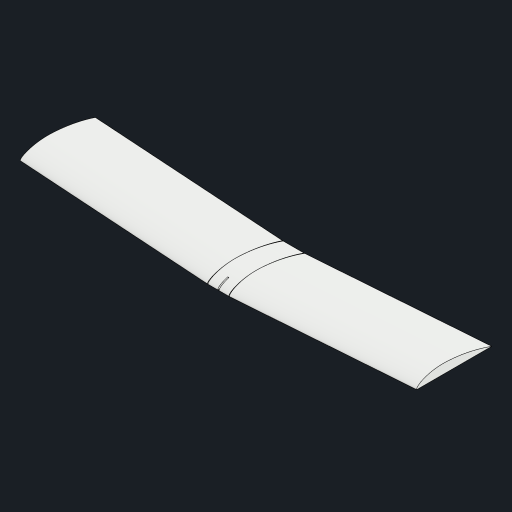
# Autodesk Inventor part: MainWing
Saved by Autodesk Inventor 2023 (Build 270158000, 158)
## iProperties
Created: 2022-05-12
Part Number: MainWing
Material: カインズの発泡スチロール
Document SubType Name: Modeling
Designer: neko2
Density: 0.02 g/cm^3
Appearance: 一般
Mass: 50.154 g
Surface Area: 3566.31 cm^2
Volume: 2507.7 cm^3
Author: neko2
Autodesk Inventor part; units mm, degrees
ref_plane "YZ Plane" through (0, 0, 0) normal (1, 0, 0) x (0, 1, 0)
ref_plane "XZ Plane" through (0, 0, 0) normal (0, 1, 0) x (-1, 0, 0)
ref_plane "XY Plane" through (0, 0, 0) normal (0, 0, 1) x (1, 0, 0)
sketch "スケッチ1" plane through (0, 0, 0) normal (1, 0, 0) x (0, 1, 0)
  spline S0 degree 3 poles (0, 0) (0.6026, 0.1485) (1.1749, 0.124) (1.7185, -0.0273) (2.4135, -0.2207) (3.0615, -0.6212) (3.65, -1.0753) (4.4423, -1.6866) (5.1266, -2.395) (5.7619, -3.1474) (6.5814, -4.1179) (7.3194, -5.1616) (8.0039, -6.2364) (8.8443, -7.5561) (9.6039, -8.9229) (10.3094, -10.317) (11.1425, -11.9631) (11.9, -13.6474) (12.5994, -15.355) (13.3997, -17.3089) (14.1237, -19.2933) (14.7857, -21.298) (15.5246, -23.5358) (16.1861, -25.7989) (16.7802, -28.0794) (17.4299, -30.5737) (17.9989, -33.0887) (18.4948, -35.618) (19.0279, -38.3372) (19.4765, -41.0727) (19.8487, -43.8185) (20.2428, -46.7262) (20.5512, -49.6454) (20.779, -52.5708) (21.0171, -55.6293) (21.1671, -58.6947) (21.2319, -61.7617) (21.2988, -64.9292) (21.2748, -68.0985) (21.1769, -71.265) (21.079, -74.4325) (20.9071, -77.5972) (20.6919, -80.7589) (20.4747, -83.9491) (20.2135, -87.1362) (19.9062, -90.3189) (19.5988, -93.503) (19.2453, -96.6827) (18.8489, -99.857) (18.4567, -102.9968) (18.0225, -106.1313) (17.5487, -109.2598) (17.0852, -112.3209) (16.5839, -115.3762) (16.0455, -118.4249) (15.525, -121.3728) (14.9697, -124.3146) (14.3808, -127.2496) (13.8184, -130.0529) (13.2253, -132.8499) (12.6033, -135.6405) (12.0172, -138.2695) (11.4054, -140.8927) (10.767, -143.5095) (10.1749, -145.936) (9.5598, -148.3569) (8.9224, -150.772) (8.342, -152.9711) (7.7431, -155.1653) (7.1255, -157.3543) (6.5752, -159.305) (6.0101, -161.2514) (5.4303, -163.1935) (4.9282, -164.8752) (4.4152, -166.5537) (3.8908, -168.2286) (3.4532, -169.6264) (3.0078, -171.0218) (2.554, -172.4145) (2.1955, -173.5145) (1.8319, -174.6128) (1.4648, -175.7099) (1.1994, -176.5028) (0.9323, -177.2952) (0.661, -178.0861) (0.497, -178.5643) (0.3315, -179.042) (0.1662, -179.5197) (0.1108, -179.6798) (0.0554, -179.8399) (0, -180) knots -1.050464 -1.050464 -1.050464 -1.050464 -1.040913 -1.040913 -1.040913 -1.028702 -1.028702 -1.028702 -1.012261 -1.012261 -1.012261 -0.991051 -0.991051 -0.991051 -0.965006 -0.965006 -0.965006 -0.934253 -0.934253 -0.934253 -0.899065 -0.899065 -0.899065 -0.859785 -0.859785 -0.859785 -0.816823 -0.816823 -0.816823 -0.770637 -0.770637 -0.770637 -0.721726 -0.721726 -0.721726 -0.670591 -0.670591 -0.670591 -0.617781 -0.617781 -0.617781 -0.564955 -0.564955 -0.564955 -0.511651 -0.511651 -0.511651 -0.458324 -0.458324 -0.458324 -0.405576 -0.405576 -0.405576 -0.353966 -0.353966 -0.353966 -0.304062 -0.304062 -0.304062 -0.2564 -0.2564 -0.2564 -0.211497 -0.211497 -0.211497 -0.169859 -0.169859 -0.169859 -0.131943 -0.131943 -0.131943 -0.098154 -0.098154 -0.098154 -0.068896 -0.068896 -0.068896 -0.044478 -0.044478 -0.044478 -0.025191 -0.025191 -0.025191 -0.011252 -0.011252 -0.011252 -0.002824 -0.002824 -0.002824 0 0 0 0
  spline S1 degree 3 poles (0, -180) (-0.1069, -180.01) (-0.1817, -179.9953) (-0.2232, -179.955) (-0.3155, -179.8653) (-0.2429, -179.6486) (-0.1926, -179.4492) (-0.0424, -178.853) (-0.0927, -178.4107) (-0.1026, -177.9372) (-0.1189, -177.1543) (-0.0246, -176.2861) (0.0432, -175.437) (0.1368, -174.2642) (0.1798, -173.1279) (0.2322, -171.9828) (0.2984, -170.5361) (0.3796, -169.0753) (0.4536, -167.6178) (0.5421, -165.8746) (0.6202, -164.136) (0.6948, -162.396) (0.7808, -160.392) (0.8622, -158.3861) (0.936, -156.3804) (1.0186, -154.1358) (1.0916, -151.8914) (1.1574, -149.6466) (1.2294, -147.1881) (1.2927, -144.7293) (1.3446, -142.2702) (1.4004, -139.6274) (1.4429, -136.9844) (1.4742, -134.3412) (1.5073, -131.5441) (1.5278, -128.7469) (1.5354, -125.9496) (1.5433, -123.0294) (1.5371, -120.1091) (1.5174, -117.189) (1.4971, -114.1787) (1.4624, -111.1684) (1.4148, -108.1584) (1.3663, -105.091) (1.3045, -102.0237) (1.2312, -98.9568) (1.1574, -95.8653) (1.0719, -92.7741) (0.9756, -89.6832) (0.8795, -86.5996) (0.7725, -83.5163) (0.666, -80.433) (0.5611, -77.3949) (0.4567, -74.3568) (0.3276, -71.3196) (0.2044, -68.4204) (0.0588, -65.5222) (-0.1152, -62.6256) (-0.2834, -59.825) (-0.4781, -57.0261) (-0.6912, -54.2286) (-0.8952, -51.5496) (-1.1161, -48.872) (-1.3464, -46.1952) (-1.5644, -43.6609) (-1.7909, -41.1273) (-2.0178, -38.5938) (-2.2298, -36.2264) (-2.4422, -33.8591) (-2.646, -31.491) (-2.8335, -29.3116) (-3.0137, -27.1314) (-3.1734, -24.9498) (-3.3176, -22.9791) (-3.4451, -21.0071) (-3.5406, -19.0332) (-3.6248, -17.293) (-3.684, -15.5514) (-3.6972, -13.8096) (-3.7085, -12.3178) (-3.6859, -10.826) (-3.5982, -9.3348) (-3.526, -8.1063) (-3.4095, -6.8782) (-3.2058, -5.6682) (-3.0458, -4.7179) (-2.8319, -3.7788) (-2.4894, -2.862) (-2.2318, -2.1725) (-1.9014, -1.4956) (-1.4256, -0.9612) (-1.0501, -0.5394) (-0.5839, -0.2064) (0, 0) knots -1.008522 -1.008522 -1.008522 -1.008522 -1.007257 -1.007257 -1.007257 -1.004442 -1.004442 -1.004442 -0.996027 -0.996027 -0.996027 -0.982114 -0.982114 -0.982114 -0.962895 -0.962895 -0.962895 -0.938614 -0.938614 -0.938614 -0.909573 -0.909573 -0.909573 -0.876126 -0.876126 -0.876126 -0.838696 -0.838696 -0.838696 -0.797703 -0.797703 -0.797703 -0.753647 -0.753647 -0.753647 -0.707026 -0.707026 -0.707026 -0.658356 -0.658356 -0.658356 -0.608182 -0.608182 -0.608182 -0.557052 -0.557052 -0.557052 -0.505513 -0.505513 -0.505513 -0.454094 -0.454094 -0.454094 -0.403429 -0.403429 -0.403429 -0.355066 -0.355066 -0.355066 -0.308307 -0.308307 -0.308307 -0.263528 -0.263528 -0.263528 -0.221134 -0.221134 -0.221134 -0.18152 -0.18152 -0.18152 -0.145062 -0.145062 -0.145062 -0.112129 -0.112129 -0.112129 -0.083096 -0.083096 -0.083096 -0.05823 -0.05823 -0.05823 -0.037743 -0.037743 -0.037743 -0.021653 -0.021653 -0.021653 -0.009552 -0.009552 -0.009552 0 0 0 0
  line L0 (0, 32.4167) -> (0, -181.4221)
  line L1 (0, -180) -> (0, -64.617)
  point P0 (0, -175.9531)
  dimension "d6" = 180
  constraints: 4 end point, 3 point on line, 1 vertical, 5 other
  measures "d6" distance of point (0, 0) L1.start
extrude "押し出し1" add sketch "スケッチ1" along normal blind 25 contours S0 L0 S1 | S1 L0 picked at (0.4314, -114.0966)
sketch "スケッチ7" plane through (25, 0, 0) normal (1, 0, 0) x (0, 0, -1)
  spline S0 degree 5 poles (180, 0) (179.1431, 0.2963) (178.2868, 0.5943) (177.4291, 0.8882) (176.5697, 1.177) (174.2182, 1.9639) (172.7247, 2.4578) (171.2286, 2.9437) (169.7297, 3.4209) (166.0631, 4.5687) (163.8927, 5.2311) (161.7177, 5.8779) (159.5382, 6.5094) (153.0432, 8.3418) (148.7151, 9.4976) (144.3716, 10.5953) (140.0126, 11.6287) (130.4, 13.7714) (125.1405, 14.8544) (119.8628, 15.8466) (114.5685, 16.7449) (105.485, 18.1203) (101.7028, 18.6441) (97.9139, 19.1179) (94.1191, 19.5393) (88.4093, 20.0906) (86.4984, 20.2611) (84.5862, 20.4181) (82.673, 20.5616) (78.8619, 20.821) (76.964, 20.9371) (75.0652, 21.0372) (73.1655, 21.1182) (69.3651, 21.2357) (67.4643, 21.2722) (65.5632, 21.2849) (63.6622, 21.272) (58.1613, 21.1559) (54.563, 20.9817) (50.9702, 20.7083) (47.3871, 20.3324) (39.2374, 19.2278) (34.6802, 18.4299) (30.1599, 17.4354) (25.6879, 16.2352) (20.0952, 14.3885) (18.8985, 13.9727) (17.7088, 13.5369) (16.5273, 13.0796) (14.3304, 12.1798) (13.3129, 11.7427) (12.3038, 11.2864) (11.3047, 10.8092) (9.4805, 9.8861) (8.6523, 9.4466) (7.8342, 8.9881) (7.0282, 8.5081) (5.5915, 7.5932) (4.956, 7.1665) (4.334, 6.7209) (3.7297, 6.2536) (2.696, 5.3807) (2.2577, 4.9848) (1.838, 4.5683) (1.4421, 4.1253) (0.8028, 3.2969) (0.5465, 2.926) (0.3215, 2.5384) (0.1434, 2.1355) (-0.0634, 1.3924) (-0.1162, 1.0576) (-0.1263, 0.714) (-0.0891, 0.3616) (0, 0) knots 0 0 0 0 0 0 0.023981 0.023981 0.023981 0.023981 0.065587 0.065587 0.065587 0.065587 0.125604 0.125604 0.125604 0.125604 0.244082 0.244082 0.244082 0.244082 0.386092 0.386092 0.386092 0.386092 0.487072 0.487072 0.487072 0.487072 0.537815 0.537815 0.537815 0.537815 0.588103 0.588103 0.588103 0.588103 0.638376 0.638376 0.638376 0.638376 0.733616 0.733616 0.733616 0.733616 0.855874 0.855874 0.855874 0.855874 0.889372 0.889372 0.889372 0.889372 0.918647 0.918647 0.918647 0.918647 0.943441 0.943441 0.943441 0.943441 0.963632 0.963632 0.963632 0.963632 0.979284 0.979284 0.979284 0.979284 0.990908 0.990908 0.990908 0.990908 1 1 1 1 1 1 projected
  line L0 (38.8422, 21.2697) -> (123.3028, 21.2697)
  line L1 (-31.0233, 21.3697) -> (204.4138, 21.3697)
  line L2 (0, 0) -> (180, 0) projected
  spline S1 degree 3 poles (0, 0) (-0.1485, 0.6026) (-0.124, 1.1749) (0.0273, 1.7185) (0.2207, 2.4135) (0.6212, 3.0615) (1.0753, 3.65) (1.6866, 4.4423) (2.395, 5.1266) (3.1474, 5.7619) (4.1179, 6.5814) (5.1616, 7.3194) (6.2364, 8.0039) (7.5561, 8.8443) (8.9229, 9.6039) (10.317, 10.3094) (11.9631, 11.1425) (13.6474, 11.9) (15.355, 12.5994) (17.3089, 13.3997) (19.2933, 14.1237) (21.298, 14.7857) (23.5358, 15.5246) (25.7989, 16.1861) (28.0794, 16.7802) (30.5737, 17.4299) (33.0887, 17.9989) (35.618, 18.4948) (38.3372, 19.0279) (41.0727, 19.4765) (43.8185, 19.8487) (46.7262, 20.2428) (49.6454, 20.5512) (52.5708, 20.779) (55.6293, 21.0171) (58.6947, 21.1671) (61.7617, 21.2319) (64.9292, 21.2988) (68.0985, 21.2748) (71.265, 21.1769) (74.4325, 21.079) (77.5972, 20.9071) (80.7589, 20.6919) (83.9491, 20.4747) (87.1362, 20.2135) (90.3189, 19.9062) (93.503, 19.5988) (96.6827, 19.2453) (99.857, 18.8489) (102.9968, 18.4567) (106.1313, 18.0225) (109.2598, 17.5487) (112.3209, 17.0852) (115.3762, 16.5839) (118.4249, 16.0455) (121.3728, 15.525) (124.3146, 14.9697) (127.2496, 14.3808) (130.0529, 13.8184) (132.8499, 13.2253) (135.6405, 12.6033) (138.2695, 12.0172) (140.8927, 11.4054) (143.5095, 10.767) (145.936, 10.1749) (148.3569, 9.5598) (150.772, 8.9224) (152.9711, 8.342) (155.1653, 7.7431) (157.3543, 7.1255) (159.305, 6.5752) (161.2514, 6.0101) (163.1935, 5.4303) (164.8752, 4.9282) (166.5537, 4.4152) (168.2286, 3.8908) (169.6264, 3.4532) (171.0218, 3.0078) (172.4145, 2.554) (173.5145, 2.1955) (174.6128, 1.8319) (175.7099, 1.4648) (176.5028, 1.1994) (177.2952, 0.9323) (178.0861, 0.661) (178.5643, 0.497) (179.042, 0.3315) (179.5197, 0.1662) (179.6798, 0.1108) (179.8399, 0.0554) (180, 0) knots -1.050464 -1.050464 -1.050464 -1.050464 -1.040913 -1.040913 -1.040913 -1.028702 -1.028702 -1.028702 -1.012261 -1.012261 -1.012261 -0.991051 -0.991051 -0.991051 -0.965006 -0.965006 -0.965006 -0.934253 -0.934253 -0.934253 -0.899065 -0.899065 -0.899065 -0.859785 -0.859785 -0.859785 -0.816823 -0.816823 -0.816823 -0.770637 -0.770637 -0.770637 -0.721726 -0.721726 -0.721726 -0.670591 -0.670591 -0.670591 -0.617781 -0.617781 -0.617781 -0.564955 -0.564955 -0.564955 -0.511651 -0.511651 -0.511651 -0.458324 -0.458324 -0.458324 -0.405576 -0.405576 -0.405576 -0.353966 -0.353966 -0.353966 -0.304062 -0.304062 -0.304062 -0.2564 -0.2564 -0.2564 -0.211497 -0.211497 -0.211497 -0.169859 -0.169859 -0.169859 -0.131943 -0.131943 -0.131943 -0.098154 -0.098154 -0.098154 -0.068896 -0.068896 -0.068896 -0.044478 -0.044478 -0.044478 -0.025191 -0.025191 -0.025191 -0.011252 -0.011252 -0.011252 -0.002824 -0.002824 -0.002824 0 0 0 0
  line L3 (180, 0) -> (0, 0) projected
  dimension "d7" = 0.1
  constraints: 4 end point, 3 horizontal, 3 horizontal alignment, 2 other
  measures "d7" distance between parallel lines of L0 L1
revolve "回転1" add sketch "スケッチ7" angle 4 about axis through (25, 21.3697, 31.0233) along (0, 0, 1)
sketch "スケッチ9" plane through (25.8095, 9.7936, -90.2873) normal (0.9975641, 0.0697565, 0) x (-0.0166942, 0.2387377, -0.9709406)
  spline S0 degree 5 poles (84.7687, -30.9516) (84.0077, -30.4588) (83.2475, -29.9646) (82.4851, -29.474) (81.7198, -28.9879) (79.6249, -27.6611) (78.2931, -26.8241) (76.9567, -25.9943) (75.6156, -25.1723) (72.3302, -23.1803) (70.3814, -22.0178) (68.4244, -20.8692) (66.4593, -19.7345) (60.5916, -16.401) (56.6659, -14.2429) (52.7114, -12.1376) (48.7263, -10.0911) (39.9059, -5.7101) (35.0584, -3.3999) (30.1715, -1.1735) (25.246, 0.9658) (16.7556, 4.4751) (13.2087, 5.8888) (9.6433, 7.2556) (6.0596, 8.573) (0.6477, 10.4747) (-1.1669, 11.0976) (-2.9859, 11.7076) (-4.8092, 12.3048) (-8.4475, 13.4688) (-10.2625, 14.0357) (-12.0821, 14.5873) (-13.9072, 15.1205) (-17.5691, 16.1442) (-19.4058, 16.6345) (-21.2487, 17.1018) (-23.0976, 17.5443) (-28.4664, 18.7479) (-32.0018, 19.4401) (-35.5557, 20.0344) (-39.1246, 20.5269) (-47.3018, 21.4048) (-51.9175, 21.7207) (-56.5445, 21.8369) (-61.1737, 21.7419) (-67.0459, 21.2873) (-68.3074, 21.17) (-69.5667, 21.0315) (-70.8233, 20.8702) (-73.1717, 20.5223) (-74.2643, 20.3415) (-75.3533, 20.14) (-76.4376, 19.9158) (-78.4296, 19.456) (-79.339, 19.2275) (-80.243, 18.9781) (-81.1404, 18.705) (-82.7544, 18.1605) (-83.4736, 17.8982) (-84.1841, 17.6144) (-84.8827, 17.3054) (-86.0953, 16.7052) (-86.6155, 16.4257) (-87.1227, 16.1218) (-87.6132, 15.7864) (-88.4321, 15.135) (-88.7698, 14.8362) (-89.0809, 14.5138) (-89.3503, 14.1652) (-89.729, 13.4932) (-89.8603, 13.1807) (-89.9523, 12.8496) (-90.0006, 12.4985) (-90.0006, 12.1261) knots 0 0 0 0 0 0 0.023981 0.023981 0.023981 0.023981 0.065587 0.065587 0.065587 0.065587 0.125604 0.125604 0.125604 0.125604 0.244082 0.244082 0.244082 0.244082 0.386092 0.386092 0.386092 0.386092 0.487072 0.487072 0.487072 0.487072 0.537815 0.537815 0.537815 0.537815 0.588103 0.588103 0.588103 0.588103 0.638376 0.638376 0.638376 0.638376 0.733616 0.733616 0.733616 0.733616 0.855874 0.855874 0.855874 0.855874 0.889372 0.889372 0.889372 0.889372 0.918647 0.918647 0.918647 0.918647 0.943441 0.943441 0.943441 0.943441 0.963632 0.963632 0.963632 0.963632 0.979284 0.979284 0.979284 0.979284 0.990908 0.990908 0.990908 0.990908 1 1 1 1 1 1 projected
  line L0 (-90.0006, 12.1261) -> (84.7687, -30.9516) projected
  point P0 (-89.5708, 13.8698)
  constraints: 1 other
extrude "押し出し3" add sketch "スケッチ9" along normal blind 450
mirror "ミラー4" about plane through (0, 10.6494, -89.9257) normal (-1, 0, 0) of "押し出し3", "押し出し1", "回転1"
sketch "スケッチ11" plane through (0, 0, 0) normal (1, 0, 0) x (0, 1, 0)
  line L0 (0, 0) -> (0.0521, 0) projected
  line L1 (0.0521, 0) -> (0.0521, -35)
  line L2 (0.0521, 0) -> (0.0521, -180) projected
  line L3 (0.0521, -35) -> (47.1624, 0)
  line L4 (47.1624, 0) -> (0.0521, 0)
  dimension "d12" = 53.39
  dimension "d13" = 35
  constraints: 6 end point, 1 perpendicular, 1 point on line
  measures "d12" angle of L3 L1
  measures "d13" distance of L0.end L1.end
extrude "押し出し4" cut sketch "スケッチ11" along normal mid plane 3
